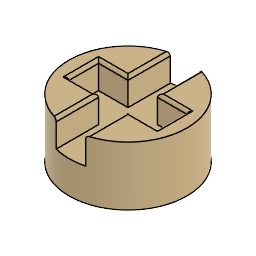
Potentiometer dial (Autodesk Fusion 360 design; units mm, degrees)
part number: 2026-06-06-23-49-45-772
Autodesk Fusion 360 part; units mm, degrees
sketch "Sketch1" plane through (0, 0, 0) normal (0, 0, 1) x (1, 0, 0)
  circle A0 centre (0, 0) radius 1
  line L0 (0.25, 0.25) -> (0.25, 0.9682)
  line L1 (0.25, -0.25) -> (0.25, -0.9682)
  line L2 (-0.25, 0.25) -> (-0.25, 0.9682)
  line L3 (-0.25, -0.25) -> (-0.25, -0.9682)
  line L4 (0.25, 0.25) -> (0.75, 0.25)
  line L5 (0.25, -0.25) -> (0.75, -0.25)
  line L6 (-0.25, -0.25) -> (-0.75, -0.25)
  line L7 (-0.25, 0.25) -> (-0.75, 0.25)
  line L8 (-0.75, -0.25) -> (-0.75, 0.25)
  line L9 (0.75, -0.25) -> (0.75, 0.25)
  constraint coincident A0.centre origin
  constraint coincident A0 L0.end
  constraint coincident A0 L1.end
  constraint coincident A0 L2.end
  constraint coincident A0 L3.end
  constraint perpendicular L0 L4
  constraint perpendicular L1 L5
extrude "Extrude2" add sketch "Sketch1" along normal blind 0.55 contours A0 L0 L1 L2 L3 L4 L5 L6 L7 L8 L9
extrude "Extrude3" add sketch "Sketch1" along normal blind 1 contours A0 L0 L1 L4 L5 L9 | A0 L2 L3 L6 L7 L8
fillet "Fillet1" radius 0.05 10 edges at (-0.5, 0.25, 1) (-0.25, 0.6091, 1) (-0.75, 0, 1) (-0.5, -0.25, 1) (-0.25, -0.6091, 1) (0.25, -0.6091, 1) (0.5, -0.25, 1) (0.5, 0.25, 1) (0.75, 0, 1) (0.25, 0.6091, 1)
